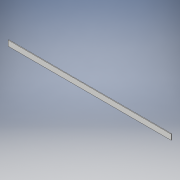
# Autodesk Inventor part: Conductive Rail
Saved by Autodesk Inventor 2018 (Build 220112000, 112)
## iProperties
Created: 2017-12-04
Part Number: Conductive Rail
Material: Generic
Document SubType Name: Modeling
Designer: Andrew
Density: 1 g/cm^3
Appearance: Default
springSteelWidth: 0.200 in
springSteelThickness: 0.026 in
Author: Andrew
Autodesk Inventor part; units mm, degrees
ref_plane "YZ Plane" through (0, 0, 0) normal (1, 0, 0) x (0, 1, 0)
ref_plane "XZ Plane" through (0, 0, 0) normal (0, 1, 0) x (-1, 0, 0)
ref_plane "XY Plane" through (0, 0, 0) normal (0, 0, 1) x (1, 0, 0)
sketch "Sketch1" plane through (0, 0, 0) normal (0, 0, 1) x (1, 0, 0)
  line L0 (-77.7875, -2.54) -> (77.7875, -2.54)
  line L1 (77.7875, -2.54) -> (77.7875, 2.54)
  line L2 (77.7875, 2.54) -> (-77.7875, 2.54)
  line L3 (-77.7875, 2.54) -> (-77.7875, -2.54)
  line L4 (-77.7875, -2.54) -> (77.7875, 2.54) construction
  line L5 (77.7875, -2.54) -> (-77.7875, 2.54) construction
  point P0 (0, 0)
  dimension "d0" = 5.08
  dimension "d1" = 155.575
  constraints: 12 end point, 2 midpoint, 2 parallel, 1 horizontal, 1 perpendicular
  measures "d0" distance of L0.end L1.end
  measures "d1" distance of L1.end L2.end
extrude "Extrusion1" add sketch "Sketch1" along normal blind 0.6548
equation "\"d0\" = springSteelWidth"
equation "\"d2\" = springSteelThickness"
equation "\"springSteelWidth\" = 5.08"
equation "\"springSteelThickness\" = 0.6548"
body "Solid1"
